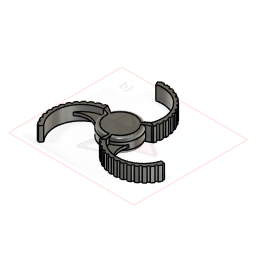
triArmWheel v1 (Autodesk Fusion 360 design; units mm, degrees)
Autodesk Fusion 360 part; units mm, degrees
note: some values were not read from the file. Set by a fixed rule: which sketch regions a step uses.
sketch "Sketch1" plane through (0, 0, 0) normal (0, 0, 1) x (1, 0, 0)
  circle A0 centre (0, 0) radius 125 construction
  dimension "d3" = 250
  constraint coincident A0.centre origin
  measures "d3" diameter of A0
sketch "Sketch2" plane through (0, 0, 0) normal (0, 0, 1) x (1, 0, 0)
  arc A0 (40, 30) -> (-37.7105, 118.6534) centre (-25.2919, 51.1533) ccw
  line L0 (-37.7105, 118.6534) -> (-34.3309, 109.2418)
  line L1 (40, 30) -> (30.9745, 34.3059)
  arc A1 (30.9745, 34.3059) -> (-34.3309, 109.2418) centre (-21.3787, 54.6052) ccw
  dimension "d4" = 10
  dimension "d5" = 10
  measures "d4" distance of A0.end L0.end
  measures "d5" distance of A0.start L1.end
extrude "Extrude1" add sketch "Sketch2" along normal blind 30 makes body 1
sketch "Sketch3" plane through (0, 0, 0) normal (1, 0, 0) x (0, 1, 0)
  line L0 (57.0602, 30) -> (57.0602, 0) construction
  line L1 (57.0602, 14) -> (34, 14) construction
  line L2 (34, 17) -> (80.1203, 17)
  line L3 (80.1203, 17) -> (80.1203, 11)
  line L4 (80.1203, 11) -> (34, 11)
  line L5 (34, 11) -> (34, 17)
  line L6 (34, 17) -> (80.1203, 11) construction
  line L7 (80.1203, 17) -> (34, 11) construction
  point P0 (57.0602, 14)
  constraint vertical L0
  constraint coincident L0 P0
  constraint perpendicular L0 L1
  constraint horizontal L2
  constraint perpendicular L2 L3
  constraint parallel L2 L4
  constraint parallel L3 L5
  constraint coincident L6 P0
  constraint coincident L7 P0
  constraint coincident P0 L1.start
extrude "Extrude2" add sketch "Sketch3" along normal blind 35 bodies 1
sketch "Sketch4" plane through (0, 0, 0) normal (0, 0, 1) x (1, 0, 0)
  arc A0 (-0.2733, 38.3918) -> (27.8716, 80.1992) centre (-6.6744, 73.0783) ccw
  line L0 (-0.2733, 38.3918) -> (-0.2733, 82.3392)
  line L1 (-0.2733, 82.3392) -> (27.8716, 80.1992)
  constraint vertical L0
extrude "Extrude3" cut sketch "Sketch4" along normal blind 20 bodies 1
sketch "Sketch5" plane through (0, 0, 0) normal (0, 0, 1) x (1, 0, 0)
  line L0 (24, 38) -> (-3.0058, 38)
  line L1 (-3.0058, 38) -> (-3.0058, 22.27)
  line L2 (-3.0058, 22.27) -> (12.1597, 14.8922)
  line L3 (12.1597, 14.8922) -> (40, 30)
  line L4 (40, 30) -> (24, 38)
  constraint horizontal L0
  constraint perpendicular L0 L1
extrude "Extrude4" add sketch "Sketch5" along normal blind 17 bodies 1
sketch "Sketch6" plane through (0, 0, 0) normal (0, 0, 1) x (1, 0, 0)
  line L0 (31, 34) -> (10, 16)
  line L1 (10, 16) -> (-3.6698, 22.3091)
  line L2 (-3.6698, 22.3091) -> (-3.6698, 38)
  line L3 (-3.6698, 38) -> (25, 38)
  line L4 (25, 38) -> (31, 35.2308)
  line L5 (31, 35.2308) -> (31, 34)
  constraint vertical L2
  constraint perpendicular L2 L3
  constraint parallel L1 L4
  constraint parallel L2 L5
extrude "Extrude5" cut sketch "Sketch6" along normal blind 11 bodies 1
copy_body "Body->Comp1" bodies 1 removing the originals makes body 2 in component "Arm"
sketch "Sketch1 (2)" plane through (0, 0, 0) normal (0, 0, 1) x (1, 0, 0) in component "Arm"
  line L0 (12, 15) -> (12, -1)
  line L1 (12, -1) -> (26, -10)
  line L2 (26, -10) -> (64.1152, 5.0873)
  line L3 (64.9788, 13.9422) -> (40, 30)
  line L4 (40, 30) -> (12, 15)
  arc A0 (64.1152, 5.0873) -> (64.9788, 13.9422) centre (62.275, 9.7363) ccw
  dimension "d16" = 5
  constraint vertical L0
  constraint parallel L1 L3
  constraint tangent L2 A0
  constraint tangent L3 A0
  measures "d16" radius of A0
extrude "Extrude1'" cut sketch "Sketch1 (2)" along normal blind 17 bodies 2 in component "Arm"
sketch "Sketch2 (2)" plane through (0, 0, 0) normal (0, 0, 1) x (1, 0, 0) in component "Arm"
  line L0 (10, 16) -> (31, 34)
  line L1 (31, 34) -> (10, 16)
  line L2 (12, 15) -> (40, 30)
  line L3 (40, 30) -> (31, 34)
  line L4 (10, 16) -> (12, 15)
  constraint coincident L0.end L1.start
  constraint coincident L0.start L1.end
extrude "Extrude2'" add sketch "Sketch2 (2)" along normal blind 30 bodies 2 in component "Arm"
sketch "Sketch3 (2)" plane through (0, 0, 30) normal (0, 0, 1) x (-1, 0, 0) in component "Arm"
  arc A0 (-40, -30) -> (37.7105, -118.6534) centre (25.2919, -51.1533) ccw
  line L0 (37.7105, -118.6534) -> (34.3309, -109.2418)
  arc A1 (-30.9745, -34.3059) -> (34.3309, -109.2418) centre (21.3787, -54.6052) ccw
  line L1 (-30.9745, -34.3059) -> (-40, -30)
  circle A2 centre (-42.0694, -38.0022) radius 2.5
  dimension "d21" = 5
  constraint coincident A0 A2.centre
  measures "d21" diameter of A2
extrude "Extrude3'" cut sketch "Sketch3 (2)" against normal blind 35 contours A0 A2 picked at (-41.2415, -38.1237) bodies 2 in component "Arm"
pattern_circular "C-Pattern1" count 36 over 360 about axis through (-25.2919, 51.1533, 0) along (0, 0, 1) of "Extrude3'" in component "Arm"
pattern_circular "C-Pattern2" count 3 over 360 about axis through (0, 0, 1.75) along (0, 0, 1) of bodies 2 makes body 3 at (-86.9197, -20.8999, 15.6667) makes body 4 at (61.5597, -64.8247, 15.6667) in component "Arm"
sketch "Sketch4 (2)" plane through (0, 0, 0) normal (0, 0, 1) x (1, 0, 0) in component "Arm"
  circle A0 centre (0, 0) radius 37.9905
  constraint coincident A0.centre origin
extrude "Extrude4'" add sketch "Sketch4 (2)" along normal blind 30 bodies 2 3 4 in component "Arm"
fillet "Fillet1" radius 7.5 tangency weight 1.68742 6 edges at (-27.1457, -26.578, 0) (-27.1457, -26.578, 30) (36.5901, -10.2199, 0) (-9.4444, 36.7979, 0) (36.5901, -10.2199, 30) (-9.4444, 36.7979, 30) on bodies 2 in component "Arm"
component "Arm" placed x (1, 0, 0) y (0, 1, 0) z (0, 0, 1) at (0, 0, 0)
named bodies: "Arm", "Arm (1)", "Arm (2)"
